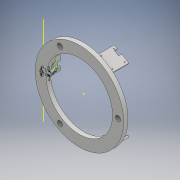
# Autodesk Inventor part: 支座
Saved by Autodesk Inventor 2017 (Build 210142000, 142)
## iProperties
Part Number: 支座
Material: 常规
Document SubType Name: Modeling
Designer: Administrator
Density: 1 g/cm^3
Appearance: 默认
Author: Administrator
Autodesk Inventor part; units mm, degrees
ref_plane "YZ Plane" through (0, 0, 0) normal (1, 0, 0) x (0, 1, 0)
ref_plane "XZ Plane" through (0, 0, 0) normal (0, 1, 0) x (-1, 0, 0)
ref_plane "XY Plane" through (0, 0, 0) normal (0, 0, 1) x (1, 0, 0)
sketch "草图1" plane through (0, 0, 0) normal (0, 1, 0) x (-1, 0, 0)
  circle A0 centre (0, 0) radius 100
  circle A1 centre (0, 0) radius 75
  dimension "d0" = 200
  dimension "d1" = 150
  constraints: 2 centre point, 2 coincident
  measures "d0" diameter of A0
  measures "d1" diameter of A1
extrude "拉伸1" add sketch "草图1" along normal blind 10
sketch "草图2" plane through (0, 10, 0) normal (0, 1, 0) x (1, 0, 0)
  line L0 (0, 0) -> (-95, 0)
  line L1 (-95, 19) -> (-95, -19)
  line L2 (-95, -19) -> (-91, -19)
  line L3 (-91, -19) -> (-91, 19)
  line L4 (-91, 19) -> (-95, 19)
  line L5 (31.0455, -91.7724) -> (63.9545, -72.7724)
  line L6 (63.9545, -72.7724) -> (61.9545, -69.3083)
  line L7 (61.9545, -69.3083) -> (29.0455, -88.3083)
  line L8 (29.0455, -88.3083) -> (31.0455, -91.7724)
  line L9 (63.9545, 72.7724) -> (31.0455, 91.7724)
  line L10 (31.0455, 91.7724) -> (29.0455, 88.3083)
  line L11 (29.0455, 88.3083) -> (61.9545, 69.3083)
  line L12 (61.9545, 69.3083) -> (63.9545, 72.7724)
  dimension "d4" = 95
  dimension "d8" = 38
  dimension "d9" = 4
  dimension "d12" = 360
  constraints: 26 end point, 2 parallel, 1 horizontal, 1 perpendicular, 1 vertical, 25 other
  measures "d4" distance of L0.start L0.end
  measures "d8" distance of L1.start L1.end
  measures "d9" distance of L2.end L1.end
extrude "拉伸2" add sketch "草图2" along normal blind 38
sketch "草图3" plane through (63.9545, 10, 72.7724) normal (0.5, 0, 0.8660254) x (0.8660254, 0, -0.5)
  line L0 (-33, 33) -> (-5, 33)
  line L1 (-5, 33) -> (-5, 5)
  line L2 (-5, 5) -> (-33, 5)
  line L3 (-33, 5) -> (-33, 33)
  line L4 (-33, 33) -> (-5, 5) construction
  line L5 (-5, 33) -> (-33, 5) construction
  circle A0 centre (-33, 33) radius 1
  circle A1 centre (-5, 33) radius 1
  circle A2 centre (-5, 5) radius 1
  circle A3 centre (-33, 4.3717) radius 1
  point P0 (-19, -10)
  point P1 (-19, 19)
  dimension "d16" = 28
  dimension "d17" = 2
  dimension "d18" = 2
  dimension "d19" = 2
  dimension "d20" = 2
  dimension "d50" = 28
  constraints: 12 end point, 4 centre point, 3 coincident, 2 midpoint, 2 parallel, 1 horizontal, 1 perpendicular, 1 other
  measures "d16" distance of L1.end L2.end
  measures "d17" diameter of A0
  measures "d18" diameter of A1
  measures "d19" diameter of A2
  measures "d20" diameter of A3
  measures "d50" distance of L0.end L1.end
extrude "拉伸3" cut sketch "草图3" against normal through all contours L3 A0 L0 | L0 A0 L3 | A1 L1 L0 | L0 L1 A1 | A3 L2 L3 | L3 L2 A3 | A2 L2 L1 | L1 L2 A2
pattern_circular "环形阵列1" count 3 over 360 about axis through (0, 0, 0) along (0, 1, 0) of "拉伸3"
sketch "草图4" plane through (-91, 10, 19) normal (1, 0, 0) x (0, 0, -1)
  line L0 (29, 29) -> (29, 0)
  line L1 (9, 0) -> (9, 29)
  line L2 (119, 0) -> (-81, 0) projected
  line L3 (26, 29) -> (26, 0)
  line L4 (26, 0) -> (12, 0)
  line L5 (12, 0) -> (12, 29)
  line L6 (29, 29) -> (29, 9)
  line L7 (9, 9) -> (9, 29)
  line L8 (9, 29) -> (12, 29)
  line L9 (26, 29) -> (29, 29)
  line L10 (9, 0) -> (12, 0)
  line L11 (26, 0) -> (29, 0)
  point P0 (19, -10)
  point P1 (19, 19)
  dimension "d26" = 20
  dimension "d28" = 14
  dimension "d29" = 20
  constraints: 22 end point, 3 horizontal, 3 parallel, 2 perpendicular, 2 point on line, 1 collinear
  measures "d26" distance of L0.end L1.start
  measures "d28" distance of L3.end L4.end
  measures "d29" distance of L0.start L6.end
sketch "草图5" plane through (0, 10, 0) normal (0, 1, 0) x (1, 0, 0)
  line L0 (-91, -10) -> (-77, -10)
  line L1 (-77, -10) -> (-77, -7)
  line L2 (-77, -7) -> (-91, -7)
  line L3 (-91, -7) -> (-91, -10)
  line L4 (-91, 10) -> (-77, 10)
  line L5 (-77, 10) -> (-77, 7)
  line L6 (-77, 7) -> (-91, 7)
  line L7 (-91, 7) -> (-91, 10)
  point P0 (0, 0)
  point P1 (-91, -10)
  point P2 (-91, 10)
  dimension "d30" = 14
  dimension "d31" = 3
  dimension "d32" = 14
  dimension "d33" = 3
  constraints: 16 end point, 4 parallel, 2 horizontal, 2 perpendicular
  measures "d30" distance of L2.end L1.end
  measures "d31" distance of L0.end L1.end
  measures "d32" distance of L5.end L6.end
  measures "d33" distance of L4.end L5.end
ref_plane "工作平面1" through (-91, 10, 10) normal (0, 0, -1) x (0, 1, 0)
ref_plane "工作平面2" through (-91, 39, -10) normal (0, 0, 1) x (0, -1, 0)
sketch "草图6" plane through (-91, 10, 10) normal (0, 0, -1) x (0, 1, 0)
  line L0 (0, 0) -> (29, 0) projected
  line L1 (0, 0) -> (0, 14) projected
  line L2 (29, 0) -> (0, 14)
  point P0 (-10, 91)
  constraints: 2 end point
extrude "拉伸4" add sketch "草图6" along normal blind 3
sketch "草图7" plane through (-91, 39, -10) normal (0, 0, 1) x (0, -1, 0)
  line L0 (0, 0) -> (29, 0) projected
  line L1 (29, 0) -> (29, 14) projected
  line L2 (0, 0) -> (29, 14)
  point P0 (39, 91)
  constraints: 2 end point
extrude "拉伸5" add sketch "草图7" along normal blind 3
pattern_circular "环形阵列2" count 3 over 360 about axis through (0, 0, 0) along (0, 1, 0) of "拉伸4", "拉伸5"
sketch "草图8" plane through (0, 10, 0) normal (0, 1, 0) x (1, 0, 0)
  circle A0 centre (87.5, 0) radius 6
  line L0 (87.5, 0) -> (0, 0)
  dimension "d41" = 12
  dimension "d42" = 87.5
  constraints: 2 end point, 1 centre point, 1 horizontal
  measures "d41" diameter of A0
  measures "d42" distance of L0.start L0.end
extrude "拉伸6" cut sketch "草图8" against normal through all
thread "螺纹1" size "M12x1.75" class "6H" standard "ANSI Metric M Profile" full length
pattern_circular "环形阵列3" count 3 over 360 about axis through (0, 0, 0) along (0, 1, 0) of "拉伸6"
sketch "草图9" plane through (-91, 10, -19) normal (1, 0, 0) x (0, 0, -1)
  line L0 (0, 38) -> (-38, 38) projected
  line L1 (-19, 38) -> (-19, 31)
  line L2 (-19, 31) -> (-8, 31)
  line L3 (-8, 31) -> (-8, 38)
  point P0 (-19, -10)
  dimension "d51" = 7
  dimension "d52" = 11
  constraints: 6 end point, 2 perpendicular, 1 midpoint, 1 point on line, 1 vertical
  measures "d51" distance of L1.start L1.end
  measures "d52" distance of L1.end L2.end
extrude "拉伸7" cut sketch "草图9" against normal through all
pattern_circular "环形阵列4" count 3 over 360 about axis through (0, 0, 0) along (0, 1, 0) of "拉伸7"
